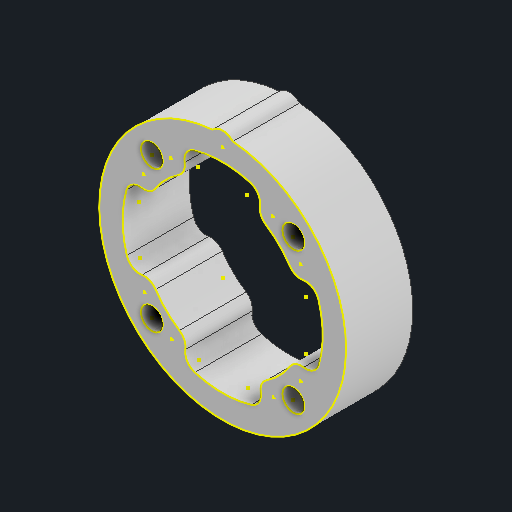
# Autodesk Inventor part: Shaft_A
Saved by Autodesk Inventor 2025.1 (Build 291241020, 241B)
## iProperties
Created: 2025-07-23
Part Number: Shaft_A
Material: 일반
Document SubType Name: Modeling
Designer: acalo
Density: 1 g/cm^3
Appearance: 기본값
Author: acalo
Autodesk Inventor part; units mm, degrees
ref_plane "YZ Plane" through (0, 0, 0) normal (1, 0, 0) x (0, 1, 0)
ref_plane "XZ Plane" through (0, 0, 0) normal (0, 1, 0) x (-1, 0, 0)
ref_plane "XY Plane" through (0, 0, 0) normal (0, 0, 1) x (1, 0, 0)
sketch "스케치1" plane through (0, 0, 0) normal (0, 0, 1) x (1, 0, 0)
  circle A0 centre (0, 0) radius 18.4
  line L0 (0, -18.4) -> (0, 19.1)
  circle A1 centre (0, 17.55) radius 1.55
  circle A2 centre (0, 0) radius 16
  circle A3 centre (0, 0) radius 12
  circle A4 centre (0, 0) radius 30 construction
  line L1 (0, 17.55) -> (0, 20.05)
  line L2 (1.4434, 20.05) -> (2.8868, 17.55)
  line L3 (2.8868, 17.55) -> (1.4434, 15.05)
  line L4 (1.4434, 15.05) -> (-1.4434, 15.05)
  line L5 (-1.4434, 15.05) -> (-2.8868, 17.55)
  line L6 (-2.8868, 17.55) -> (-1.4434, 20.05)
  line L7 (-1.4434, 20.05) -> (1.4434, 20.05)
  point P0 (-2.494, 18.2302)
  point P1 (2.494, 18.2302)
  point P2 (1.3263, 18.3521)
  point P3 (-1.3263, 18.3521)
  dimension "d0" = 36.8
  dimension "d2" = 3.1
  dimension "d1" = 37.5
  dimension "d3" = 32
  dimension "d4" = 24
  dimension "d5" = 60
  dimension "d6" = 2.5
  constraints: 16 end point, 5 coincident, 3 centre point, 2 point on line, 1 midpoint, 1 vertical, 19 other
  measures "d1" distance of L0.start L0.end
  measures "d3" diameter of A2
  measures "d4" diameter of A3
  measures "d5" diameter of A4
  measures "d6" distance of L1.start L1.end
extrude "돌출1" add sketch "스케치1" along normal blind 4 contours L0 A2 L3 L2 A0 | A0 L6 L5 A2 L0 | A2 L5 L4 L0 A3 | L0 A3 L4 L3 A2
extrude "돌출2" add sketch "스케치1" against normal blind 10 contours L0 A2 L3 L2 A0 | A0 L6 L5 A2 L0 | A0 A1 A2 L5 L6 | A2 L5 L4 L0 A3 | L0 A3 L4 L3 A2 | L2 L3 A2 A1 A0 | A2 L0 L4 L5 | A2 L3 L4 L0
sketch "스케치2" plane through (0, 0, 4) normal (0, 0, 1) x (1, 0, 0)
  line L0 (0, 0) -> (10.6066, 10.6066)
  line L1 (0, 0) -> (15, 0) construction
  circle A0 centre (10.6066, 10.6066) radius 1.65
  circle A1 centre (-14.4889, 3.8823) radius 1.65
  circle A2 centre (3.8823, -14.4889) radius 1.65
  dimension "d11" = 15
  dimension "d12" = 45
  dimension "d13" = 3.3
  dimension "d16" = 360
  constraints: 4 end point, 3 centre point, 1 coincident, 1 equal length, 1 horizontal, 7 other
  measures "d11" distance of L0.start L0.end
  measures "d12" angle of L1 L0
  measures "d13" diameter of A0
extrude "돌출3" cut sketch "스케치2" against normal through all
sketch "스케치3" plane through (0, 0, -10) normal (0, 0, -1) x (-1, 0, 0)
  circle A0 centre (14.4889, 3.8823) radius 1.65 projected
  line L0 (11.7005, 4.6294) -> (13.7417, 6.6707)
  line L1 (13.7417, 6.6707) -> (16.5301, 5.9235)
  line L2 (17.2773, 3.1351) -> (15.236, 1.0939)
  line L3 (15.236, 1.0939) -> (12.4476, 1.841)
  arc A1 (-1.3263, 18.3521) -> (1.3263, 18.3521) centre (0, 0) ccw projected
  circle A2 centre (0, 0) radius 12 projected
  line L4 (17.3447, 6.1418) -> (16.5301, 5.9235)
  line L5 (11.7005, 4.6294) -> (11.1334, 4.4775)
  line L6 (18.0918, 3.3534) -> (17.2773, 3.1351)
  line L7 (12.4476, 1.841) -> (11.8805, 1.6891)
  line L8 (-11.3537, 13.395) -> (-8.5654, 12.6478)
  line L9 (-11.9501, 13.9913) -> (-11.3537, 13.395)
  line L10 (-7.8182, 9.8595) -> (-7.4031, 9.4443)
  line L11 (-8.5654, 12.6478) -> (-7.8182, 9.8595)
  line L12 (-9.8595, 7.8182) -> (-12.6478, 8.5654)
  line L13 (-9.8595, 7.8182) -> (-9.4443, 7.4031)
  line L14 (-12.6478, 8.5654) -> (-13.395, 11.3537)
  line L15 (-13.9913, 11.9501) -> (-13.395, 11.3537)
  line L16 (-5.9235, -16.5301) -> (-6.6707, -13.7417)
  line L17 (-6.1418, -17.3447) -> (-5.9235, -16.5301)
  line L18 (-4.6294, -11.7005) -> (-4.4775, -11.1334)
  line L19 (-6.6707, -13.7417) -> (-4.6294, -11.7005)
  line L20 (-1.841, -12.4476) -> (-1.0939, -15.236)
  line L21 (-1.841, -12.4476) -> (-1.6891, -11.8805)
  line L22 (-1.0939, -15.236) -> (-3.1351, -17.2773)
  line L23 (-3.3534, -18.0918) -> (-3.1351, -17.2773)
  dimension "d23" = 360
  constraints: 48 end point, 4 point on circle, 55 other
extrude "돌출4" [suppressed]
fillet "모깎기1" radius 0.6 4 edges at (-1.3263, 18.3521, -5) (1.3263, 18.3521, -5) (2.494, 18.2302, 2) (-2.494, 18.2302, 2)
sketch "스케치4" plane through (0, 0, 4) normal (0, 0, 1) x (1, 0, 0)
  arc A0 (2.219, 18.2657) -> (1.5476, 17.6366) centre (2.1466, 17.6701) ccw
  arc A1 (-1.5476, 17.6366) -> (1.5476, 17.6366) centre (0, 17.55) ccw
  arc A2 (-1.5476, 17.6366) -> (-2.219, 18.2657) centre (-2.1466, 17.6701) ccw
  arc A3 (-2.219, 18.2657) -> (-3.5967, 18.045) centre (0, 0) ccw projected
  arc A4 (-2.8868, 17.55) -> (-3.5967, 18.045) centre (-3.4794, 17.4566) ccw projected
  line L0 (-1.4434, 15.05) -> (-2.8868, 17.55) projected
  line L1 (1.4434, 15.05) -> (-1.4434, 15.05) projected
  line L2 (2.8868, 17.55) -> (1.4434, 15.05)
  arc A5 (3.5967, 18.045) -> (2.8868, 17.55) centre (3.4794, 17.4566) ccw
  arc A6 (3.5967, 18.045) -> (-2.219, 18.2657) centre (0, 0) ccw
  line L3 (0, 17.55) -> (0, 17.35)
  arc A7 (-3.5967, 18.045) -> (3.5967, 18.045) centre (0, 0) ccw projected
  line L4 (0, -18.4) -> (0, 19.2)
  circle A8 centre (0, 17.35) radius 1.85
  point P0 (1.5671, 18.3331)
  point P1 (-1.5671, 18.3331)
  point P2 (-2.219, 18.2657)
  dimension "d28" = 0.2
  dimension "d29" = 37.6
  constraints: 13 point on circle, 11 centre point, 6 end point, 2 vertical, 1 coincident, 3 other
  measures "d28" distance of L3.start L3.end
  measures "d29" distance of L4.start L4.end
extrude "돌출5" add sketch "스케치4" against normal up to surface (14 mm away) contours A6 A5 L2 L1 L4 A8 A0 | A0 A8 A6 | A8 L4 A1 A0 | A0 A1 L4 L3 A6 A8 | A6 L4 A8 | L4 L3 A1 A2 A8 A6 | A6 A8 L4 | L4 A8 A2 A1 | L4 L1 L0 A4 A3 A2 A8 | A8 A2 A6
sketch "스케치5" plane through (0, 0, 4) normal (0, 0, 1) x (1, 0, 0)
  circle A0 centre (0, 0) radius 19.4
  arc A1 (-1.4847, 18.34) -> (1.4847, 18.34) centre (0, 0) ccw
  circle A2 centre (0, 17) radius 2
  line L0 (0, 0) -> (0, 7.8398)
  line L1 (0, -18.4) -> (0, 19)
  arc A3 (1.5671, 18.3331) -> (-1.5671, 18.3331) centre (0, 17.35) ccw
  point P0 (0, 3.9199)
  dimension "d32" = 38.8
  dimension "d35" = 37.4
  dimension "d36" = 4
  constraints: 10 point on circle, 4 centre point, 4 end point, 2 vertical, 1 coincident, 1 midpoint, 1 other
  measures "d32" diameter of A0
  measures "d35" distance of L1.start L1.end
  measures "d36" diameter of A2
extrude "돌출6" cut sketch "스케치5" against normal through all contours A1 A3 A2
sketch "스케치6" plane through (0, 0, 4) normal (0, 0, 1) x (1, 0, 0)
  circle A0 centre (0, 0) radius 19.4
  dimension "d39" = 38.8
  constraints: 1 centre point, 1 coincident
  measures "d39" diameter of A0
sketch "스케치7" plane through (0, 0, 4) normal (0, 0, 1) x (1, 0, 0)
  circle A0 centre (0, 0) radius 12 projected
  circle A1 centre (0, 0) radius 15
  line L0 (0, 0) -> (6.3393, 13.5946)
  line L1 (0, 0) -> (15, 0) construction
  line L2 (0, 0) -> (-12.2873, 8.6036)
  line L3 (0, 0) -> (15, 0) construction
  line L4 (0, 0) -> (-14.9429, -1.3073)
  line L5 (0, 0) -> (-1.3073, -14.9429)
  line L6 (0, 0) -> (8.6036, -12.2873)
  line L7 (0, 0) -> (13.5946, 6.3393)
  point P0 (10.8757, 5.0714)
  point P1 (6.8829, -9.8298)
  point P2 (-1.0459, -11.9543)
  point P3 (-11.9543, -1.0459)
  point P4 (-9.8298, 6.8829)
  point P5 (5.0714, 10.8757)
  dimension "d40" = 3
  dimension "d41" = 65
  dimension "d42" = 145
  dimension "d45" = 360
  constraints: 16 end point, 2 equal length, 2 horizontal, 2 point on circle, 1 centre point, 16 other
  measures "d40" radial gap between concentric circles of A0 A1
  measures "d41" angle of L1 L0
  measures "d42" angle of L3 L2
extrude "돌출7" cut sketch "스케치7" against normal through all contours A0 L7 A1 L6 | A0 L2 A1 L0 | L5 A1 L4 A0
fillet "모깎기2" radius 2 18 edges at (-9.8298, 6.8829, 2) (-9.8298, 6.8829, -5) (-11.9543, -1.0459, 2) (-11.9543, -1.0459, -5) (6.3393, 13.5946, -3) (10.8757, 5.0714, 2) (10.8757, 5.0714, -5) (5.0714, 10.8757, 2) (5.0714, 10.8757, -5) (13.5946, 6.3393, -3) (6.8829, -9.8298, 2) (6.8829, -9.8298, -5) (8.6036, -12.2873, -3) (-1.0459, -11.9543, 2) (-1.0459, -11.9543, -5) (-1.3073, -14.9429, -3) (-14.9429, -1.3073, -3) (-12.2873, 8.6036, -3)
sketch "스케치8" plane through (0, 0, 4) normal (0, 0, 1) x (1, 0, 0)
  arc A0 (14.3668, 4.3123) -> (14.408, -4.1723) centre (0, 0) ccw
  arc A1 (-13.3149, -1.1021) -> (-14.5981, -3.4488) centre (-12.6517, -2.989) ccw
  arc A2 (-13.3149, -1.1021) -> (-11.9811, 0.6726) centre (-13.978, 0.7847) ccw
  arc A3 (-10.7123, 5.4081) -> (-11.9811, 0.6726) centre (0, 0) ccw
  arc A4 (-10.7123, 5.4081) -> (-10.9799, 7.6119) centre (-12.4977, 6.3094) ccw
  arc A5 (-10.9179, 10.2859) -> (-10.9799, 7.6119) centre (-9.4622, 8.9144) ccw
  arc A6 (4.1723, 14.408) -> (-10.9179, 10.2859) centre (0, 0) ccw
  arc A7 (5.5852, 12.137) -> (4.1723, 14.408) centre (3.616, 12.487) ccw
  arc A8 (5.5852, 12.137) -> (6.4751, 10.1031) centre (7.5543, 11.787) ccw
  arc A9 (10.0397, 6.5731) -> (6.4751, 10.1031) centre (0, 0) ccw
  arc A10 (10.0397, 6.5731) -> (12.0821, 5.7029) centre (11.7129, 7.6686) ccw
  arc A11 (14.3668, 4.3123) -> (12.0821, 5.7029) centre (12.4512, 3.7373) ccw
  arc A12 (10.2859, -10.9179) -> (14.3668, 4.3123) centre (0, 0) ccw
  arc A13 (7.6119, -10.9799) -> (10.2859, -10.9179) centre (8.9144, -9.4622) ccw
  arc A14 (7.6119, -10.9799) -> (5.4081, -10.7123) centre (6.3094, -12.4977) ccw
  arc A15 (0.6726, -11.9811) -> (5.4081, -10.7123) centre (0, 0) ccw
  arc A16 (0.6726, -11.9811) -> (-1.1021, -13.3149) centre (0.7847, -13.978) ccw
  arc A17 (-3.4488, -14.5981) -> (-1.1021, -13.3149) centre (-2.989, -12.6517) ccw
  circle A18 centre (3.8823, -14.4889) radius 1.65
  circle A19 centre (-14.4889, 3.8823) radius 1.65
  circle A20 centre (10.6066, 10.6066) radius 1.65
  arc A21 (-1.4847, 18.34) -> (1.4847, 18.34) centre (0, 0) ccw
  arc A22 (1.4847, 18.34) -> (-1.4847, 18.34) centre (0, 17) ccw
  arc A23 (-12.137, 5.5852) -> (-10.1031, 6.4751) centre (-11.787, 7.5543) ccw
  arc A24 (-6.5731, 10.0397) -> (-10.1031, 6.4751) centre (0, 0) ccw
  arc A25 (-6.5731, 10.0397) -> (-5.7029, 12.0821) centre (-7.6686, 11.7129) ccw
  arc A26 (-4.3123, 14.3668) -> (-5.7029, 12.0821) centre (-3.7373, 12.4512) ccw
  circle A27 centre (-10.6066, 10.6066) radius 1.65
  arc A28 (-12.137, 5.5852) -> (-14.408, 4.1723) centre (-12.487, 3.616) ccw
  arc A29 (-5.5852, -12.137) -> (-6.4751, -10.1031) centre (-7.5543, -11.787) ccw
  arc A30 (-10.0397, -6.5731) -> (-6.4751, -10.1031) centre (0, 0) ccw
  arc A31 (-10.0397, -6.5731) -> (-12.0821, -5.7029) centre (-11.7129, -7.6686) ccw
  arc A32 (-14.3668, -4.3123) -> (-12.0821, -5.7029) centre (-12.4512, -3.7373) ccw
  circle A33 centre (-10.6066, -10.6066) radius 1.65
  arc A34 (-5.5852, -12.137) -> (-4.1723, -14.408) centre (-3.616, -12.487) ccw
  arc A35 (12.137, -5.5852) -> (10.1031, -6.4751) centre (11.787, -7.5543) ccw
  arc A36 (6.5731, -10.0397) -> (10.1031, -6.4751) centre (0, 0) ccw
  arc A37 (6.5731, -10.0397) -> (5.7029, -12.0821) centre (7.6686, -11.7129) ccw
  arc A38 (4.3123, -14.3668) -> (5.7029, -12.0821) centre (3.7373, -12.4512) ccw
  circle A39 centre (10.6066, -10.6066) radius 1.65
  arc A40 (12.137, -5.5852) -> (14.408, -4.1723) centre (12.487, -3.616) ccw
  point P0 (-9.3775, 11.7074)
  point P1 (-11.4438, 9.1848)
  point P2 (-10.5208, 6.0061)
  point P3 (6.0692, -10.5121)
  point P4 (9.1848, -11.4438)
  point P5 (11.7074, -9.3775)
  point P6 (-11.7074, -9.3775)
  point P7 (-9.3775, -11.7074)
  point P8 (-4.1723, -14.408)
  point P9 (5.3183, -13.6762)
  point P10 (2.2674, -14.8276)
  point P11 (-14.8276, 2.2674)
  point P12 (-13.6041, 5.275)
  dimension "d52" = 360
  constraints: 80 centre point, 68 point on circle, 85 other
extrude "돌출8" add sketch "스케치8" against normal blind 10 contours A26 A25 A24 A23 A4 A5 A27 A0 | A19 A28 A0 | A0 A19 | A0 A39 A13 A14 A37 A36 A35 A40 | A32 A31 A30 A29 A34 A0 A33 | A18 A0 | A0 A38 A18 picked at (-13.9781, 5.1348) picked at (5.1735, -13.9875)
extrude "돌출9" cut sketch "스케치8" against normal blind 10 contours A0 A27 | A5 A27 A0 | A28 A23 A4 A3 A2 A1 A0 A19 | A39 A0 | A0 A39 A13 | A0 A33 | A37 A38 A18 A0 A17 A16 A15 A14 picked at (-11.4742, 9.5269) picked at (9.5268, -11.4741) picked at (-10.9907, -10.9907)
thicken "두껍게 하기1" operation cut thickness 4 both sides no extend neighbours no toward (0, 0, 1) faces at (0, 17.9905, -10) (1.9175, 16.5112, -10)
thicken "두껍게 하기2" operation add thickness 0.1 both sides no extend neighbours no toward (-0.1623091, 0.98674, 0) faces at (-2.9865, 18.156, 1.3333) (-1.7847, 18.3132, -0.6667) (6.4878, 17.2183, 2.6667) (-1.5488, 18.3347, -2.6667) (1.7847, 18.3132, -0.6667) (1.503, 18.3385, -2.6667) (-2.9865, 18.156, -2) (2.5265, 18.2257, -2) (-0.0797, 18.9984, -2.6667)
sketch "스케치9" plane through (0, 0, 4) normal (0, 0, 1) x (1, 0, 0)
  arc A0 (-1.5318, 18.4365) -> (1.5318, 18.4365) centre (0, 0) ccw projected
  arc A1 (1.5318, 18.4365) -> (-1.5318, 18.4365) centre (0, 17) ccw projected
  circle A2 centre (10.6066, -10.6066) radius 1.65 projected
  circle A3 centre (-10.6066, 10.6066) radius 1.65 projected
  arc A4 (-12.137, 5.5852) -> (-14.408, 4.1723) centre (-12.487, 3.616) ccw projected
  arc A5 (-12.137, 5.5852) -> (-10.1031, 6.4751) centre (-11.787, 7.5543) ccw projected
  arc A6 (-6.5731, 10.0397) -> (-10.1031, 6.4751) centre (0, 0) ccw projected
  arc A7 (-6.5731, 10.0397) -> (-5.7029, 12.0821) centre (-7.6686, 11.7129) ccw projected
  arc A8 (-4.3123, 14.3668) -> (-5.7029, 12.0821) centre (-3.7373, 12.4512) ccw projected
  arc A9 (4.1723, 14.408) -> (-4.3123, 14.3668) centre (0, 0) ccw projected
  arc A10 (5.5852, 12.137) -> (4.1723, 14.408) centre (3.616, 12.487) ccw projected
  arc A11 (5.5852, 12.137) -> (6.4751, 10.1031) centre (7.5543, 11.787) ccw projected
  arc A12 (10.0397, 6.5731) -> (6.4751, 10.1031) centre (0, 0) ccw projected
  arc A13 (10.0397, 6.5731) -> (12.0821, 5.7029) centre (11.7129, 7.6686) ccw projected
  arc A14 (14.3668, 4.3123) -> (12.0821, 5.7029) centre (12.4512, 3.7373) ccw projected
  arc A15 (14.408, -4.1723) -> (14.3668, 4.3123) centre (0, 0) ccw projected
  arc A16 (12.137, -5.5852) -> (14.408, -4.1723) centre (12.487, -3.616) ccw projected
  arc A17 (12.137, -5.5852) -> (10.1031, -6.4751) centre (11.787, -7.5543) ccw projected
  arc A18 (6.5731, -10.0397) -> (10.1031, -6.4751) centre (0, 0) ccw projected
  arc A19 (6.5731, -10.0397) -> (5.7029, -12.0821) centre (7.6686, -11.7129) ccw projected
  arc A20 (4.3123, -14.3668) -> (5.7029, -12.0821) centre (3.7373, -12.4512) ccw projected
  arc A21 (-4.1723, -14.408) -> (4.3123, -14.3668) centre (0, 0) ccw projected
  arc A22 (-5.5852, -12.137) -> (-4.1723, -14.408) centre (-3.616, -12.487) ccw projected
  arc A23 (-5.5852, -12.137) -> (-6.4751, -10.1031) centre (-7.5543, -11.787) ccw projected
  arc A24 (-10.0397, -6.5731) -> (-6.4751, -10.1031) centre (0, 0) ccw projected
  arc A25 (-10.0397, -6.5731) -> (-12.0821, -5.7029) centre (-11.7129, -7.6686) ccw projected
  arc A26 (-14.3668, -4.3123) -> (-12.0821, -5.7029) centre (-12.4512, -3.7373) ccw projected
  arc A27 (-14.408, 4.1723) -> (-14.3668, -4.3123) centre (0, 0) ccw projected
  circle A28 centre (-10.6066, -10.6066) radius 1.65 projected
  circle A29 centre (10.6066, 10.6066) radius 1.65 projected
